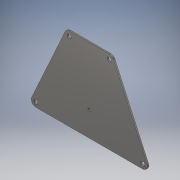
# Autodesk Inventor part: Frame
Saved by Autodesk Inventor 2019 (Build 230136000, 136)
## iProperties
Created: 2019-08-25
Part Number: Frame
Material: Steel, Mild
Document SubType Name: Modeling
Designer: DIBYOJYOTI
Density: 7.85 g/cm^3
Appearance: Semi-Polished
Mass: 482.281 g
Surface Area: 330.942 cm^2
Volume: 61.4371 cm^3
Author: DIBYOJYOTI
Autodesk Inventor part; units mm, degrees
ref_plane "YZ Plane" through (0, 0, 0) normal (1, 0, 0) x (0, 1, 0)
ref_plane "XZ Plane" through (0, 0, 0) normal (0, 1, 0) x (-1, 0, 0)
ref_plane "XY Plane" through (0, 0, 0) normal (0, 0, 1) x (1, 0, 0)
sketch "Sketch1" plane through (0, 0, 0) normal (0, 0, 1) x (1, 0, 0)
  circle A0 centre (50, 110) radius 3
  circle A1 centre (0, 0) radius 3
  circle A2 centre (160, 0) radius 3
  circle A3 centre (80, 30) radius 2.05
  arc A4 (50, 117) -> (43.6274, 112.8966) centre (50, 110) ccw
  circle A5 centre (110, 110) radius 3
  arc A6 (116.3726, 112.8966) -> (110, 117) centre (110, 110) ccw
  arc A7 (-6.3726, 2.8966) -> (0, -7) centre (0, 0) ccw
  arc A8 (160, -7) -> (166.3726, 2.8966) centre (160, 0) ccw
  line L0 (-6.3726, 2.8966) -> (43.6274, 112.8966)
  line L1 (50, 117) -> (110, 117)
  line L2 (166.3726, 2.8966) -> (116.3726, 112.8966)
  line L3 (0, -7) -> (160, -7)
  dimension "d7" = 6
  dimension "d9" = 6
  dimension "d10" = 6
  dimension "d11" = 4.1
  dimension "d12" = 14
  dimension "d13" = 6
  dimension "d14" = 14
  dimension "d15" = 14
  dimension "d16" = 14
  dimension "d25" = 160
  dimension "d26" = 60
  dimension "d27" = 110
  dimension "d28" = 30
  constraints: 9 centre point, 8 end point, 8 point on circle, 7 tangent, 5 coincident
  measures "d7" diameter of A0
  measures "d9" diameter of A1
  measures "d10" diameter of A2
  measures "d11" diameter of A3
  measures "d12" diameter of A4
  measures "d13" diameter of A5
  measures "d14" diameter of A6
  measures "d15" diameter of A7
  measures "d16" diameter of A8
  measures "d25" distance of A8.centre point (0, 0)
  measures "d26" distance of A5.centre A0.centre
  measures "d27" vertical distance of A2.centre A5.centre
  measures "d28" vertical distance of A8.centre A3.centre
extrude "Extrusion1" add sketch "Sketch1" along normal blind 2
body "Solid1"
